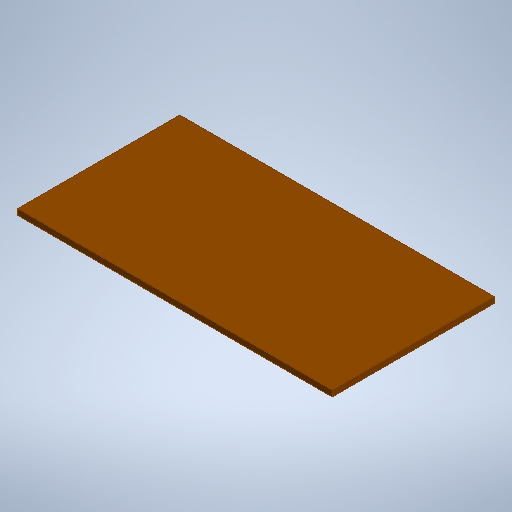
# Autodesk Inventor part: Plywood Board
Saved by Autodesk Inventor 2025.1 (Build 291241000, 241)
## iProperties
Category: <PART CATAGORY>
Created: 2025-03-03
Part Number: Plywood Board
Material: Plywood, Finish
Document SubType Name: Modeling
Designer: chowg
Mass: 22.4007 g
Surface Area: 285.27 cm^2
Volume: 40.581 cm^3
Density: 0.552 g/cm^3
Appearance: Plywood - New
Title: <TITLE>
Author: chowg
Revision Number: 1
Autodesk Inventor part; units mm, degrees
ref_plane "YZ Plane" through (0, 0, 0) normal (1, 0, 0) x (0, 1, 0)
ref_plane "XZ Plane" through (0, 0, 0) normal (0, 1, 0) x (-1, 0, 0)
ref_plane "XY Plane" through (0, 0, 0) normal (0, 0, 1) x (1, 0, 0)
sketch "Sketch6" plane through (0, 0, 0) normal (0, 0, 1) x (1, 0, 0)
  point P0 (0, 0)
sketch "Sketch7" plane through (0, 0, 0) normal (0, 0, 1) x (1, 0, 0)
  line L0 (0, 0) -> (0, 3)
  line L1 (0, 0) -> (3, 0) construction
  line L2 (0, 3) -> (162, 3)
  line L3 (162, 3) -> (162, 0)
  line L4 (162, 0) -> (0, 0)
  dimension "d85" = 3
  dimension "d86" = 90
  dimension "d87" = 162
  dimension "d88" = 3
  dimension "d89" = 90
  constraints: 10 end point, 3 perpendicular, 1 horizontal, 1 vertical
  measures "d85" distance of L0.start L0.end
  measures "d86" angle of L1 L0
  measures "d87" distance of L0.end L2.end
  measures "d88" distance of L2.end L3.end
  measures "d89" angle of L2 L3
extrude "Extrusion3" add sketch "Sketch7" along normal blind 83.5
body "Solid2"
